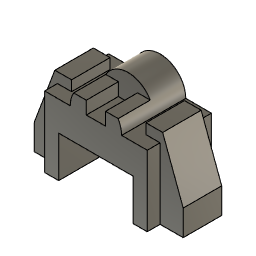
Sketch11_Final v1 (Autodesk Fusion 360 design; units mm, degrees)
Autodesk Fusion 360 part; units mm, degrees
sketch "Sketch1" plane through (0, 0, 0) normal (0, 1, 0) x (1, 0, 0)
  line L0 (29, 0) -> (40, 0)
  line L1 (40, 0) -> (40, -55)
  line L2 (40, -55) -> (20, -55)
  line L3 (0, -55) -> (0, -32)
  line L4 (0, -70) -> (0, -85)
  line L5 (0, -35) -> (0, -32)
  line L6 (-29, 0) -> (-40, 0)
  line L7 (-40, 0) -> (-40, -55)
  line L8 (-40, -55) -> (-20, -55)
  line L9 (29, 0) -> (29, -32)
  line L10 (29, -32) -> (0, -32)
  line L11 (-29, -32) -> (0, -32)
  line L12 (-29, 0) -> (-29, -32)
  arc A0 (-20, -55) -> (20, -55) centre (0, -55) ccw
  dimension "d1" = 40
  dimension "d2" = 55
  dimension "d3" = 29
  dimension "d4" = 32
  dimension "d5" = 40
  constraint horizontal L0
  constraint vertical L1
  constraint horizontal L2
  constraint vertical L3
  constraint vertical L4
  constraint symmetric L0.end L4 L6.end
  constraint symmetric L1.end L4 L7.end
  constraint vertical L9
  constraint horizontal L10
  constraint symmetric L4 L0.start L6.start
  constraint symmetric L4 L9.end L11.start
  constraint symmetric L4 L3.end L5.end
  constraint coincident L3 L5.start
  measures "d1" distance of origin L0.end
  measures "d2" distance of origin L3.start
  measures "d3" distance of origin L0.start
  measures "d4" distance of origin L3.end
  measures "d5" diameter of A0
extrude "Extrude1" add sketch "Sketch1" along normal mid plane 50
sketch "Sketch2" plane through (0, 0, 32) normal (0, 0, -1) x (1, 0, 0)
  line L0 (-29, 25) -> (-29, -25)
  line L1 (-29, -25) -> (29, -25)
  line L2 (29, -25) -> (29, 25)
  line L3 (29, 25) -> (-29, 25)
  line L4 (40, 15) -> (27, 15)
  line L5 (27, 15) -> (27, -15)
  line L6 (27, -15) -> (40, -15)
  line L7 (40, 15) -> (58, 15)
  line L8 (58, 15) -> (58, -15)
  line L9 (58, -15) -> (40, -15)
  line L10 (0, -35) -> (0, -40)
  line L11 (-58, -15) -> (-40, -15)
  line L12 (-27, -15) -> (-40, -15)
  line L13 (-27, 15) -> (-27, -15)
  line L14 (-40, 15) -> (-27, 15)
  line L15 (-40, 15) -> (-58, 15)
  line L16 (-58, 15) -> (-58, -15)
  dimension "d9" = 13
  dimension "d10" = 30
  dimension "d11" = 18
  dimension "d12" = 30
  constraint horizontal L4
  constraint vertical L5
  constraint horizontal L6
  constraint horizontal L7
  constraint vertical L8
  constraint horizontal L9
  constraint vertical L10
  constraint symmetric L4.start L10 L14.start
  constraint symmetric L4.end L10 L13.start
  constraint symmetric L5.end L10 L12.start
  constraint symmetric L6.end L10 L11.end
  constraint symmetric L7.end L10 L15.end
  constraint symmetric L8.end L10 L11.start
  measures "d9" distance of L4.start L4.end
  measures "d10" distance of L4.start L6.end
  measures "d11" distance of L4.start L7.end
  measures "d12" distance of L4.start L6.end
extrude "Extrude2" add sketch "Sketch2" against normal blind 63 from surface at 32 contours L0 L11 L12 L14 L15 L16 | L2 L4 L6 L7 L8 L9
sketch "Sketch3" plane through (0, 0, 0) normal (0, 1, 0) x (1, 0, 0)
  line L0 (-7.5, -65) -> (-7.5, -55)
  line L1 (7.5, -55) -> (7.5, -65)
  line L2 (-7.5, -55) -> (7.5, -55)
  line L3 (0, -85) -> (0, -96)
  line L4 (-57.9919, -20) -> (-42, -62.9941)
  line L5 (-42, -62.9941) -> (-63.2403, -5.8898)
  line L6 (-63.2403, -5.8898) -> (-39.5238, -69.6512)
  line L7 (-39.5238, -69.6512) -> (-63.2403, -69.6512)
  line L8 (-63.2403, -69.6512) -> (-63.2403, -5.8898)
  line L9 (39.5238, -69.6512) -> (63.2403, -69.6512)
  line L10 (63.2403, -5.8898) -> (39.5238, -69.6512)
  line L11 (63.2403, -69.6512) -> (63.2403, -5.8898)
  line L12 (-7.5, -65) -> (-20, -65)
  line L13 (7.5, -65) -> (20.2492, -65)
  arc A0 (-20, -65) -> (20.2492, -65) centre (0.1246, -54.9377) ccw
  dimension "d24" = 45
  constraint parallel L0 L1
  constraint vertical L3
  constraint parallel L4 L5
  constraint parallel L5 L6
  constraint symmetric L3 L5.end L10.start
  constraint symmetric L3 L6.end L9.start
  constraint symmetric L3 L7.end L9.end
  constraint perpendicular L0 L12
  constraint perpendicular L1 L13
  measures "d24" diameter of A0
extrude "Extrude3" cut sketch "Sketch3" along normal mid plane 70 contours L4 L5 L6 L7 L8 | L9 L10 L11
extrude "Extrude4" cut sketch "Sketch3" against normal blind 30 contours L0 L1 L2 L12 L13 A0
